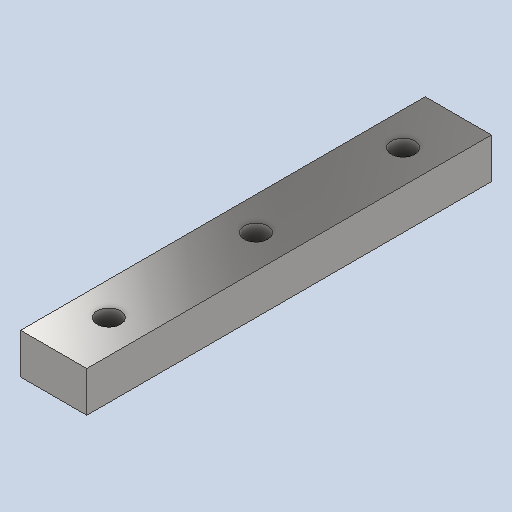
# Autodesk Inventor part: TH22_slider_95
Saved by Autodesk Inventor 2022 (Build 260153000, 153)
## iProperties
Created: 2021-11-11
Part Number: TH22_slider_95
Material: 鉄、可鍛鉄
Document SubType Name: Modeling
Designer: 中島 青蔵
Density: 7.15 g/cm^3
Appearance: 半つや出し
Author: 中島 青蔵
Autodesk Inventor part; units mm, degrees
ref_plane "YZ Plane" through (0, 0, 0) normal (1, 0, 0) x (0, 1, 0)
ref_plane "XZ Plane" through (0, 0, 0) normal (0, 1, 0) x (-1, 0, 0)
ref_plane "XY Plane" through (0, 0, 0) normal (0, 0, 1) x (1, 0, 0)
sketch "スケッチ1" plane through (0, 0, 0) normal (0, 0, 1) x (1, 0, 0)
  line L0 (0, 0) -> (9, 0)
  line L1 (9, 0) -> (9, 5.5)
  line L2 (9, 5.5) -> (0, 5.5)
  line L3 (0, 5.5) -> (0, 0)
  dimension "d0" = 9
  dimension "d1" = 5.5
  constraints: 8 end point
  measures "d0" distance of L2.end L1.end
  measures "d1" distance of L1.end L0.end
extrude "押し出し1" add sketch "スケッチ1" along normal blind 55
sketch "スケッチ2" plane through (0, 5.5, 0) normal (0, 1, 0) x (1, 0, 0)
  line L0 (9, 0) -> (0, 0) projected
  point P0 (4.5, -7.5)
  point P1 (4.5, -27.5)
  point P2 (4.5, -47.5)
  point P3 (4.5, -67.5)
  point P4 (4.5, -87.5)
  dimension "d4" = 7.5
  dimension "d5" = 20
  dimension "d6" = 20
  dimension "d7" = 20
  dimension "d8" = 20
  measures "d4" distance from line of L0 point (4.5, -7.5)
  measures "d5" distance of point (4.5, -7.5) point (4.5, -27.5)
  measures "d6" distance of point (4.5, -27.5) point (4.5, -47.5)
  measures "d7" distance of point (4.5, -47.5) point (4.5, -67.5)
  measures "d8" distance of point (4.5, -67.5) point (4.5, -87.5)
hole "穴1" at (4.5, 5.5, 7.5) at (4.5, 5.5, 27.5) at (4.5, 5.5, 47.5) at (4.5, 5.5, 67.5) at (4.5, 5.5, 87.5) direction (0, -1, 0) diameter 3.2 end through all
equation "\"d6\" = d5"
equation "\"d7\" = d5"
equation "\"d8\" = d5"
